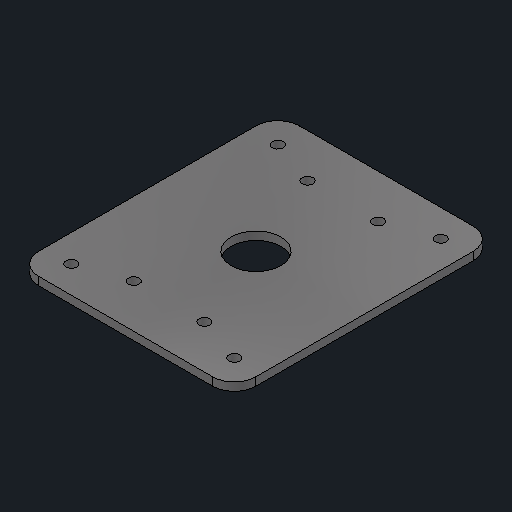
# Autodesk Inventor part: Gooseneck Model-2 Sheet-1
Saved by Autodesk Inventor 2025.1 (Build 291241000, 241)
## iProperties
RuleStatus: InUse
Created: 2026-02-16
Part Number: Gooseneck Model-2 Sheet-1
User Status: Released
Material: SS304
Document SubType Name: Sheet Metal
Designer: Desktop -24
Density: 7.99949 g/cm^3
Sheet Metal Rule: 3/8" (3.150 Die)
Appearance: Semi-Polished(1)
AfterDocNew0: Mat. Selection
encoded128: ÌStandard Î
encoded39: *STANDARD*
Family: SS304
Author: Desktop -24
Revision Number: 0
Autodesk Inventor part; units mm, degrees
ref_plane "YZ Plane" through (0, 0, 0) normal (1, 0, 0) x (0, 1, 0)
ref_plane "XZ Plane" through (0, 0, 0) normal (0, 1, 0) x (-1, 0, 0)
ref_plane "XY Plane" through (0, 0, 0) normal (0, 0, 1) x (1, 0, 0)
sketch "Sketch4" plane through (0, 0, 0) normal (0, 1, 0) x (-1, 0, 0)
  line L0 (-127, 152.4) -> (127, 152.4)
  line L1 (127, 152.4) -> (127, -152.4)
  line L2 (127, -152.4) -> (-127, -152.4)
  line L3 (-127, -152.4) -> (-127, 152.4)
  line L4 (-127, 152.4) -> (127, -152.4) construction
  line L5 (127, 152.4) -> (-127, -152.4) construction
  point P0 (0, 0)
  dimension "d6" = 304.8
  dimension "d7" = 254
  measures "d6" distance of L0.end L1.end
  measures "d7" distance of L1.end L2.end
extrude "Plate1" add sketch "Sketch4" against normal blind 9.525
sketch "Sketch6" plane through (0, 0, 0) normal (0, 1, 0) x (1, 0, 0)
  circle A0 centre (0, 0) radius 29.083
  dimension "d19" = 58.166
  constraints: 1 centre point, 1 coincident
  measures "d19" diameter of A0
extrude "Cut1" cut sketch "Sketch6" against normal blind 9.525
sketch "Sketch7" plane through (0, 0, 0) normal (0, 1, 0) x (1, 0, 0)
  line L0 (-41.275, -101.6) -> (41.275, -101.6)
  line L1 (41.275, -101.6) -> (41.275, 101.6)
  line L2 (41.275, 101.6) -> (-41.275, 101.6)
  line L3 (-41.275, 101.6) -> (-41.275, -101.6)
  line L4 (-41.275, -101.6) -> (41.275, 101.6) construction
  line L5 (41.275, -101.6) -> (-41.275, 101.6) construction
  line L6 (127, 152.4) -> (-127, 152.4) projected
  point P0 (0, 0)
  point P1 (112.6998, 215.9)
  point P2 (-112.6998, 215.9)
  point P3 (-127, 152.4)
  dimension "d22" = 82.55
  dimension "d23" = 50.8
  constraints: 12 end point, 2 midpoint, 2 parallel, 1 horizontal, 1 perpendicular, 1 other
  measures "d22" distance of L1.end L2.end
hole "Hole1" at (-41.275, 0, 101.6) at (41.275, 0, 101.6) at (-41.275, 0, -101.6) at (41.275, 0, -101.6) direction (0, -1, 0) diameter 12.7 depth 9.525
sketch "Sketch8" plane through (0, 0, 0) normal (0, 1, 0) x (1, 0, 0)
  line L0 (-95.25, -120.65) -> (95.25, -120.65)
  line L1 (95.25, -120.65) -> (95.25, 120.65)
  line L2 (95.25, 120.65) -> (-95.25, 120.65)
  line L3 (-95.25, 120.65) -> (-95.25, -120.65)
  line L4 (-95.25, -120.65) -> (95.25, 120.65) construction
  line L5 (95.25, -120.65) -> (-95.25, 120.65) construction
  line L6 (127, -152.4) -> (127, 152.4) projected
  line L7 (127, 152.4) -> (-127, 152.4) projected
  point P0 (0, 0)
  dimension "d32" = 31.75
  dimension "d33" = 31.75
  constraints: 12 end point, 2 midpoint, 2 parallel, 1 horizontal, 1 perpendicular
  measures "d32" distance between parallel lines of L6 L1
  measures "d33" distance between parallel lines of L2 L7
hole "Hole2" at (95.25, 0, 120.65) at (95.25, 0, -120.65) at (-95.25, 0, -120.65) at (-95.25, 0, 120.65) direction (0, -1, 0) diameter 12.7 depth 9.525
fillet "Corner Round2" radius 25.4 4 edges at (127, -4.7625, 152.4) (127, -4.7625, -152.4) (-127, -4.7625, 152.4) (-127, -4.7625, -152.4)
equation "\"d20\" = Thickness"
equation "\"d29\" = Thickness"
equation "\"d39\" = Thickness"
equation "\"d8\" = Thickness"
equation "\"BendReliefWidth\" = Thickness"
equation "\"BendReliefDepth\" = 0.5 * Thickness"
equation "\"CornerReliefSize\" = 4 * Thickness"
equation "\"MinimumRemnant\" = 2 * Thickness"
equation "\"TransitionRadius\" = BendRadius"
equation "\"JacobiRadiusSize\" = Thickness"
equation "\"GapSize\" = Thickness"
equation "\"Thickness\" = 9.525"
equation "\"BendRadius\" = 13.208"
body "Solid4"
